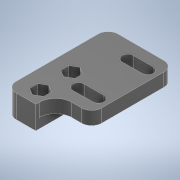
# Autodesk Inventor part: shoulder endstop support
Saved by Autodesk Inventor 2022 (Build 260153000, 153)
## iProperties
Created: 2022-03-29
Part Number: shoulder endstop support
Material: Genérico
Document SubType Name: Modeling
Designer: JK
Density: 1 g/cm^3
Appearance: Suave - Negro
Author: JK
Autodesk Inventor part; units mm, degrees
ref_plane "YZ Plane" through (0, 0, 0) normal (1, 0, 0) x (0, 1, 0)
ref_plane "XZ Plane" through (0, 0, 0) normal (0, 1, 0) x (-1, 0, 0)
ref_plane "XY Plane" through (0, 0, 0) normal (0, 0, 1) x (1, 0, 0)
sketch "Boceto1" plane through (0, 0, 0) normal (0, 1, 0) x (-1, 0, 0)
  line L0 (18.3407, 8.3801) -> (-1.6593, 8.3801)
  line L1 (-1.6593, 8.3801) -> (-1.6593, -16.6199)
  line L2 (-1.6593, -16.6199) -> (18.3407, -16.6199)
  line L3 (18.3407, -16.6199) -> (18.3407, 8.3801)
  circle A0 centre (1.3407, 3.3801) radius 1.7
  circle A1 centre (1.3407, -11.6199) radius 1.7
  circle A2 centre (7.3407, -11.6199) radius 1.7
  circle A3 centre (7.3407, 3.3801) radius 1.7
  line L4 (7.3407, -13.3199) -> (1.3407, -13.3199)
  line L5 (1.3407, -13.3199) -> (1.3407, -9.9199)
  line L6 (1.3407, -9.9199) -> (7.3407, -9.9199)
  line L7 (7.3407, -9.9199) -> (7.3407, -13.3199)
  line L8 (7.3407, 1.6801) -> (1.3407, 1.6801)
  line L9 (1.3407, 1.6801) -> (1.3407, 5.0801)
  line L10 (1.3407, 5.0801) -> (7.3407, 5.0801)
  line L11 (7.3407, 5.0801) -> (7.3407, 1.6801)
  point P0 (0, 0)
  point P1 (7.3407, 3.3801)
  point P2 (1.3407, -13.3199)
  point P3 (1.3407, 1.6801)
  dimension "d0" = 3.4
  dimension "d1" = 3
  dimension "d2" = 5
  dimension "d3" = 15
  dimension "d6" = 25
  dimension "d16" = 20
  dimension "d17" = 6
  constraints: 24 end point, 9 horizontal, 6 parallel, 3 perpendicular, 2 midpoint, 2 point on line, 2 tangent, 2 vertical alignment, 1 centre point, 10 other
  measures "d0" diameter of A0
  measures "d1" distance from line of A0.centre L1
  measures "d2" distance from line of L2 point (1.341, -11.62)
  measures "d3" distance of point (1.341, -11.62) A0.centre
  measures "d6" distance of L2.end L0.start
  measures "d16" distance of L1.end L2.end
  measures "d17" distance of L4.start L4.end
extrude "Extrusión1" add sketch "Boceto1" along normal blind 4
sketch "Boceto2" plane through (0, 4, 0) normal (0, 1, 0) x (1, 0, 0)
  line L0 (1.6593, 16.6199) -> (-18.3407, 16.6199) projected
  line L1 (-18.3407, -8.3801) -> (1.6593, -8.3801) projected
  line L2 (-18.3407, 16.6199) -> (-9.3407, 16.6199)
  line L3 (-9.3407, 16.6199) -> (-9.3407, -8.3801)
  line L4 (-9.3407, -8.3801) -> (-18.3407, -8.3801)
  line L5 (-18.3407, -8.3801) -> (-18.3407, 16.6199)
  point P0 (0, 0)
  point P1 (-9.3407, 16.6199)
  dimension "d7" = 9
  constraints: 8 end point, 2 parallel, 1 horizontal, 1 perpendicular, 1 point on line
  measures "d7" distance between parallel lines of L3 L5
extrude "Extrusión2" add sketch "Boceto2" against normal blind 7
sketch "Boceto5" plane through (0, -3, 0) normal (0, -1, 0) x (1, 0, 0)
  line L0 (-9.3407, 8.3801) -> (-18.3407, 8.3801) projected
  line L1 (-18.3407, 8.3801) -> (-9.3407, 8.3801)
  line L2 (-9.3407, 8.3801) -> (-9.3407, 14.3801)
  line L3 (-9.3407, 14.3801) -> (-18.3407, 14.3801)
  line L4 (-18.3407, 14.3801) -> (-18.3407, 8.3801)
  line L5 (-9.3407, -16.6199) -> (-9.3407, 8.3801) projected
  point P0 (0, 0)
  point P1 (-9.3407, 8.3801)
  dimension "d24" = 6
  constraints: 8 end point, 2 parallel, 1 collinear, 1 horizontal, 1 perpendicular
  measures "d24" distance of L3.end L0.end
extrude "Extrusión5" add sketch "Boceto5" against normal up to surface (7 mm away)
fillet "Empalme2" radius 5 1 edges at (-9.3407, 2, 8.3801)
sketch "Boceto3" plane through (0, -3, 0) normal (0, -1, 0) x (1, 0, 0)
  circle A0 centre (-12.3407, 9.8801) radius 1.2
  circle A1 centre (-12.3407, 0.3801) radius 1.2
  line L0 (-9.3407, -16.6199) -> (-9.3407, 8.3801) projected
  line L1 (-18.3407, -16.6199) -> (-9.3407, -16.6199) projected
  line L2 (-18.3407, 14.3801) -> (-18.3407, -16.6199) projected
  point P0 (0, 0)
  dimension "d10" = 2.4
  dimension "d11" = 9.5
  dimension "d19" = 17
  dimension "d30" = 6
  constraints: 2 centre point, 1 equal radius, 1 vertical alignment
  measures "d10" diameter of A0
  measures "d11" distance of A0.centre A1.centre
  measures "d19" distance from line of L1 A1.centre
  measures "d30" distance from line of L2 A0.centre
extrude "Extrusión3" cut sketch "Boceto3" against normal through all
sketch "Boceto4" plane through (0, 4, 0) normal (0, 1, 0) x (1, 0, 0)
  circle A0 centre (-12.3407, -9.8801) radius 1.2 projected
  circle A1 centre (-12.3407, -9.8801) radius 2.15
  line L0 (-12.3407, -12.3627) -> (-14.4907, -11.1214)
  line L1 (-14.4907, -11.1214) -> (-14.4907, -8.6388)
  line L2 (-14.4907, -8.6388) -> (-12.3407, -7.3975)
  line L3 (-12.3407, -7.3975) -> (-10.1907, -8.6388)
  line L4 (-10.1907, -8.6388) -> (-10.1907, -11.1214)
  line L5 (-10.1907, -11.1214) -> (-12.3407, -12.3627)
  circle A2 centre (-12.3407, -0.3801) radius 1.2 projected
  circle A3 centre (-12.3407, -0.3801) radius 2.15
  line L6 (-12.3407, 2.1025) -> (-10.1907, 0.8612)
  line L7 (-10.1907, 0.8612) -> (-10.1907, -1.6214)
  line L8 (-10.1907, -1.6214) -> (-12.3407, -2.8627)
  line L9 (-12.3407, -2.8627) -> (-14.4907, -1.6214)
  line L10 (-14.4907, -1.6214) -> (-14.4907, 0.8612)
  line L11 (-14.4907, 0.8612) -> (-12.3407, 2.1025)
  point P0 (0, 0)
  dimension "d29" = 4.3
  constraints: 24 end point, 4 coincident, 2 centre point, 2 tangent, 1 equal radius, 1 vertical, 1 vertical alignment, 26 other
  measures "d29" diameter of A1
extrude "Extrusión4" cut sketch "Boceto4" against normal blind 5 contours A0 | A1 | L4 L5 A1 | A1 L3 L4 | A1 L2 L3 | L5 L0 A1 | A1 L1 L2 | L0 L1 A1 | A2 | A3 | L7 L8 A3 | A3 L6 L7 | A3 L11 L6 | L8 L9 A3 | A3 L10 L11 | L9 L10 A3
fillet "Empalme3" radius 3 4 edges at (-18.3407, 0.5, 14.3801) (-18.3407, 0.5, -16.6199) (1.6593, 2, 8.3801) (1.6593, 2, -16.6199)
sketch "Boceto6" plane through (0, 0, 0) normal (0, -1, 0) x (1, 0, 0)
  point P0 (0, 0)
sketch "Boceto7" plane through (0, -3, 0) normal (0, -1, 0) x (1, 0, 0)
  arc A0 (-7.3407, 5.0801) -> (-7.3407, 1.6801) centre (-7.3407, 3.3801) ccw projected
  circle A1 centre (-7.3407, 3.3801) radius 3
  arc A2 (-7.3407, -9.9199) -> (-7.3407, -13.3199) centre (-7.3407, -11.6199) ccw projected
  circle A3 centre (-7.3407, -11.6199) radius 3
  point P0 (0, 0)
  dimension "d31" = 6
  dimension "d32" = 6
  constraints: 2 centre point, 2 coincident
  measures "d31" diameter of A1
  measures "d32" diameter of A3
extrude "Extrusión6" cut sketch "Boceto7" against normal up to surface (3 mm away)
